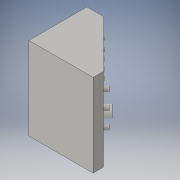
# Autodesk Inventor part: genral outlines
Saved by Autodesk Inventor 2016 (Build 200138000, 138)
## iProperties
Created: 2016-05-17
Part Number: genral outlines
Material: Generic
Document SubType Name: Modeling
Designer: Lillahunden
Density: 1 g/cm^3
Appearance: Default
Author: Lillahunden
Autodesk Inventor part; units mm, degrees
ref_plane "YZ Plane" through (0, 0, 0) normal (1, 0, 0) x (0, 1, 0)
ref_plane "XZ Plane" through (0, 0, 0) normal (0, 1, 0) x (-1, 0, 0)
ref_plane "XY Plane" through (0, 0, 0) normal (0, 0, 1) x (1, 0, 0)
sketch "Sketch1" plane through (0, 0, 0) normal (0, 0, 1) x (1, 0, 0)
  line L0 (0, 0) -> (155, 0)
  line L1 (155, 0) -> (155, 25)
  line L2 (155, 25) -> (40, 140)
  line L3 (40, 140) -> (0, 140)
  line L4 (0, 140) -> (0, 0)
  dimension "d4" = 40
  dimension "d5" = 140
  dimension "d10" = 25
  dimension "d13" = 45
  constraints: 11 end point, 2 perpendicular, 1 horizontal, 1 parallel
  measures "d4" distance of L2.end L3.end
  measures "d5" distance of L0.start L3.end
  measures "d10" distance of L0.end L1.end
  measures "d13" angle of L1 L2
extrude "Extrusion1" add sketch "Sketch1" along normal blind 200
sketch "Sketch2" plane through (40, 140, 0) normal (0.7071, 0.7071, 0) x (-0.7071, 0.7071, 0)
  circle A0 centre (-34.3317, 177.5117) radius 2.5
  point P0 (-70.7107, 0)
  dimension "d9" = 5
  constraints: 1 centre point
  measures "d9" diameter of A0
extrude "Extrusion2" add sketch "Sketch2" along normal blind 2
pattern_linear "Rectangular Pattern1" count 5 spacing 20 along (0, 0, -1) count 2 spacing 35 along (0.7071, -0.7071, 0) of "Extrusion2"
sketch "Sketch3" plane through (40, 140, 0) normal (0.7071, 0.7071, 0) x (-0.7071, 0.7071, 0)
  circle A0 centre (-54.6677, 40.8266) radius 12.5
  point P0 (-70.7107, 0)
  dimension "d20" = 25
  constraints: 1 centre point
  measures "d20" diameter of A0
extrude "Extrusion3" add sketch "Sketch3" along normal blind 15
sketch "Sketch4" plane through (40, 140, 0) normal (0.7071, 0.7071, 0) x (-0.7071, 0.7071, 0)
  circle A0 centre (-132.1111, 141.7709) radius 5
  point P0 (-70.7107, 0)
  dimension "d23" = 10
  constraints: 1 centre point
  measures "d23" diameter of A0
extrude "Extrusion4" add sketch "Sketch4" along normal blind 10
pattern_linear "Rectangular Pattern2" count 3 spacing 40 along (0, 0, -1) of "Extrusion4"
body "Solid1"
